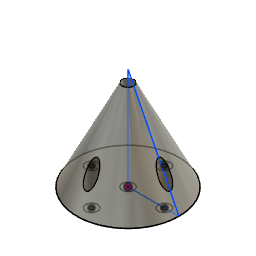
_base_mount.aa962479-57d6-4ac7-87ad-e300ce6e1ebd (Autodesk Fusion 360 design; units mm, degrees)
Autodesk Fusion 360 part; units mm, degrees
note: some values were not read from the file. Set by a fixed rule: which sketch regions a step uses.
sketch "Sketch1" plane through (0, 0, 0) normal (0, 1, 0) x (1, 0, 0)
  circle A0 centre (0, 0) radius 35
  circle A1 centre (25, 0) radius 1.5
  line L0 (0, 0) -> (25, 0)
  circle A2 centre (0, 25) radius 1.5
  circle A3 centre (-25, 0) radius 1.5
  circle A4 centre (0, -25) radius 1.5
  circle A5 centre (0, 0) radius 4
  circle A6 centre (-25, 0) radius 4
  circle A7 centre (0, 25) radius 4
  circle A8 centre (25, 0) radius 4
  circle A9 centre (0, -25) radius 4
  dimension "d1" = 70
  dimension "d2" = 3
  dimension "d3" = 25
  dimension "d5" = 360
  dimension "d6" = 8
  dimension "d21" = 8
  dimension "d22" = 8
  dimension "d23" = 8
  dimension "d24" = 8
  measures "d1" diameter of A0
  measures "d2" diameter of A1
  measures "d3" distance of A0.centre A1.centre
  measures "d6" diameter of A5
  measures "d21" diameter of A6
  measures "d22" diameter of A7
  measures "d23" diameter of A8
  measures "d24" diameter of A9
sketch "Sketch3" plane through (0, 0, 0) normal (0, 0, 1) x (1, 0, 0)
  line L0 (0, 0) -> (0, 70)
  line L1 (0, 0) -> (35, 0)
  line L2 (35, 0) -> (0, 70)
  dimension "d18" = 70
  dimension "d19" = 35
  measures "d18" distance of L0.start L0.end
  measures "d19" distance of L0.start L1.end
revolve "Revolve1" add sketch "Sketch3" angle 360 about axis through (0, 0, 0) along (0, 1, 0)
extrude "Extrude4" add sketch "Sketch1" along normal blind 7 contours A5
extrude "Extrude6" cut sketch "Sketch1" along normal blind 30 contours A1 | A2 | A3 | A4 | A6 | A7 | A8 | A9
extrude "Extrude7" add sketch "Sketch1" along normal blind 7 contours A6 | A7 | A8 | A9
extrude "Extrude8" cut sketch "Sketch1" along normal blind 70 contours A5
extrude "Extrude9" add sketch "Sketch1" along normal blind 1 contours A5
sketch "Sketch4" plane through (0, 0, 0) normal (0, 0, 1) x (1, 0, 0)
